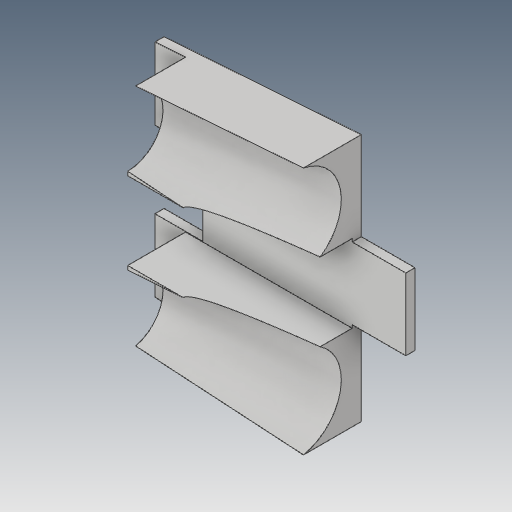
# Autodesk Inventor part: hand-palm
Saved by Autodesk Inventor 2018 (Build 220112000, 112)
## iProperties
Created: 2019-04-01
Part Number: hand-palm
Material: Generic
Document SubType Name: Modeling
Designer: Tsche
Density: 1 g/cm^3
Appearance: Default
Author: Tsche
Autodesk Inventor part; units mm, degrees
ref_plane "YZ Plane" through (0, 0, 0) normal (1, 0, 0) x (0, 1, 0)
ref_plane "XZ Plane" through (0, 0, 0) normal (0, 1, 0) x (-1, 0, 0)
ref_plane "XY Plane" through (0, 0, 0) normal (0, 0, 1) x (1, 0, 0)
sketch "Sketch2" plane through (0, 0, 0) normal (0, 0, 1) x (1, 0, 0)
  line L0 (0, -57.05) -> (0, 57.05) construction
  line L1 (-56.66, 0) -> (58.56, 0) construction
  line L2 (-24.5, 0) -> (-24.5, -12.575)
  line L3 (-24.5, -12.575) -> (-40.2, -12.575)
  line L4 (-40.2, -12.575) -> (-40.2, -36.2257)
  line L5 (-40.2, -36.2257) -> (24.5, -40.75)
  line L6 (24.5, -40.75) -> (24.5, -11.75)
  line L7 (24.5, -11.75) -> (42.1, -11.75)
  line L8 (42.1, -11.75) -> (42.1, 0)
  line L9 (-24.5, 0) -> (-24.5, 12.575)
  line L10 (-24.5, 12.575) -> (-40.2, 12.575)
  line L11 (-40.2, 12.575) -> (-40.2, 36.2257)
  line L12 (-40.2, 36.2257) -> (24.5, 40.75)
  line L13 (24.5, 40.75) -> (24.5, 11.75)
  line L14 (24.5, 11.75) -> (42.1, 11.75)
  line L15 (42.1, 11.75) -> (42.1, 0)
  line L16 (-35, 12.575) -> (-35, -12.575) construction
  line L17 (35, 11.75) -> (35, -11.75) construction
  point P0 (0, 0)
  dimension "d0" = 25.15
  dimension "d1" = 70
  dimension "d2" = 10.5
  dimension "d3" = 10.5
  dimension "d4" = 5.2
  dimension "d5" = 7.1
  dimension "d6" = 23.5
  dimension "d7" = 81.5
  dimension "d8" = 8
  constraints: 32 end point, 6 point on line, 6 symmetric about line, 5 perpendicular, 1 vertical, 1 other
  measures "d0" distance between parallel lines of L3 L10
  measures "d1" distance between parallel lines of L17 L16
  measures "d2" distance between parallel lines of L2 L16
  measures "d3" distance between parallel lines of L17 L6
  measures "d4" distance between parallel lines of L16 L4
  measures "d5" distance between parallel lines of L8 L17
  measures "d6" distance between parallel lines of L7 L14
  measures "d7" distance of L5.end L12.end
  measures "d8" angle of L12 L5
extrude "Extrusion1" add sketch "Sketch2" along normal blind 3
fillet "Fillet1" [suppressed]
sketch "Sketch3" plane through (0, 0, 3) normal (0, 0, 1) x (1, 0, 0)
  line L0 (-30.15, -25.625) -> (24.5, -25.625) construction
  line L1 (24.5, -40.75) -> (24.5, -11.75) construction
  line L2 (-40.2, -36.2257) -> (24.5, -40.75) construction
  line L3 (-40.2, -12.575) -> (-40.2, -36.2257) construction
  line L4 (-24.5, -12.575) -> (-40.2, -12.575) construction
  line L5 (24.5, -12.75) -> (-30.15, -12.75)
  line L6 (-30.15, -12.75) -> (-30.15, -36.9285)
  line L7 (-30.15, -36.9285) -> (24.5, -40.75)
  line L8 (24.5, -12.75) -> (24.5, -40.75)
  point P0 (0, 0)
  dimension "d12" = 25.625
  dimension "d13" = 28
  dimension "d14" = 54.65
  constraints: 10 end point, 4 point on line, 2 collinear, 2 perpendicular, 1 horizontal
  measures "d12" distance from line of point (0, 0) L0
  measures "d13" distance from line of L1.start L5
  measures "d14" distance between parallel lines of L1 L6
extrude "Extrusion2" add sketch "Sketch3" along normal blind 19
sketch "Sketch4" plane through (0, 0, 22) normal (0, 0, 1) x (1, 0, 0)
  line L0 (-30.15, -25.625) -> (24.5, -25.625) construction
  line L1 (-30.15, -36.9285) -> (24.5, -40.75) construction
  line L2 (-30.15, -12.75) -> (-30.15, -36.9285) projected
  line L3 (24.5, -40.75) -> (24.5, -12.75) projected
  line L4 (-30.15, -25.625) -> (24.5, -25.625)
  line L5 (-30.15, -36.9285) -> (-30.15, -37.2292)
  line L6 (-30.15, -37.2292) -> (24.5, -41.0507)
  line L7 (24.5, -41.0507) -> (24.5, -40.75)
  point P0 (0, 0)
  dimension "d18" = 0.3
  constraints: 8 end point, 2 equal length, 2 vertical
  measures "d18" distance between parallel lines of L6 L1
revolve "Revolution1" cut sketch "Sketch4" angle 360 about axis through (-30.15, -25.625, 22) along (1, 0, 0)
mirror "Mirror1" about plane through (0, 0, 0) normal (0, 1, 0) of "Extrusion2", "Revolution1"
equation "\"d0\" = finger_width + 2 * finger_link_clearence"
equation "\"d12\" = 0.5 * dist_hinge_points"
equation "\"finger_width\" = 25"
equation "\"finger_thickness\" = 8"
equation "\"finger_part_A_length\" = 42.8625"
equation "\"finger_part_B_length\" = 28.575"
equation "\"finger_link_width\" = 3.5"
equation "\"finger_link_clearence\" = 0.075"
equation "\"tol\" = 0.5 * finger_link_clearence"
equation "\"link_tol\" = 0.254"
equation "\"bore_press\" = 2.925"
equation "\"bore_clearance\" = 3.025"
equation "\"bar_diameter\" = 6.5"
equation "\"bar_thickness\" = 4"
equation "\"bar_width\" = 7"
equation "\"hinge_dist_sym_plane\" = 4"
equation "\"hinge_thickness\" = 3"
equation "\"hinge_act_length_c\" = 7.62"
equation "\"hinge_act_length_bc\" = 16.66875"
equation "\"hinge_act_length_ab\" = 11.049"
equation "\"hinge_act_length_a\" = 21.43125"
equation "\"hinge_guid_length_c\" = 9.525"
equation "\"hinge_guid_length_bc\" = 9.525"
equation "\"hinge_guid_length_ab\" = 17.145"
equation "\"hinge_guid_length_a\" = 17.145"
equation "\"bar_length_bc\" = finger_part_B_length"
equation "\"bar_act_length_ab\" = 40.48125"
equation "\"bar_guid_length_ab\" = 43.275"
equation "\"champfer\" = 0.3"
equation "\"fillet\" = 0.4"
equation "\"gear_diameter\" = 14"
equation "\"dist_finger_BC\" = 56.5"
equation "\"hinge_point\" = 15"
equation "\"dist_hinge_points\" = 51.25"
body "Solid1"
